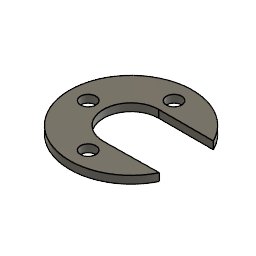
Practice Design from Txt Book (Autodesk Fusion 360 design; units mm, degrees)
part number: 2026-05-18-22-26-25-394
Autodesk Fusion 360 part; units mm, degrees
sketch "Sketch1" plane through (0, 0, 0) normal (0, 1, 0) x (1, 0, 0)
  line L0 (0, 18) -> (35.7211, 18)
  line L1 (0, -18) -> (35.9683, -17.5009)
  arc A0 (35.7211, 18) -> (35.9683, -17.5009) centre (0, 0) ccw
  arc A1 (0, 18) -> (0.4995, -17.9931) centre (0, 0) ccw
  circle A2 centre (0, 28) radius 5
  circle A3 centre (0, -28) radius 5
  circle A4 centre (-28, 0) radius 5
  dimension "d1" = 80
  dimension "d2" = 36
  dimension "d4" = 28
  dimension "d5" = 28
  dimension "d6" = 28
  dimension "d7" = 10
  dimension "d8" = 10
  dimension "d9" = 10
  constraint coincident A0.centre A1.centre
  constraint concentric A0 A1
  constraint horizontal L0
  constraint coincident L1.start A1
  constraint coincident L1 A1.end
  measures "d1" diameter of A0
  measures "d2" diameter of A1
  measures "d4" distance of A0.centre A2.centre
  measures "d5" distance of A0.centre A4.centre
  measures "d6" distance of A0.centre A3.centre
  measures "d7" diameter of A2
  measures "d8" diameter of A3
  measures "d9" diameter of A4
extrude "Extrude1" add sketch "Sketch1" along normal blind 5
